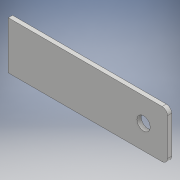
# Autodesk Inventor part: ramie3
Saved by Autodesk Inventor 2017.3 (Build 213256000, 256)
## iProperties
Created: 2019-03-17
Part Number: ramie3
Material: Ogólny
Document SubType Name: Modeling
Designer: legox
Density: 1 g/cm^3
Appearance: Domyślna
Author: legox
Autodesk Inventor part; units mm, degrees
ref_plane "YZ Plane" through (0, 0, 0) normal (1, 0, 0) x (0, 1, 0)
ref_plane "XZ Plane" through (0, 0, 0) normal (0, 1, 0) x (-1, 0, 0)
ref_plane "XY Plane" through (0, 0, 0) normal (0, 0, 1) x (1, 0, 0)
sketch "Szkic1" plane through (0, 0, 0) normal (0, 1, 0) x (-1, 0, 0)
  line L0 (2, 0) -> (60, 0)
  line L1 (60, 0) -> (60, -18)
  line L2 (60, -18) -> (2, -18)
  line L3 (0, -16) -> (0, -2)
  circle A0 centre (9, -9) radius 2.5
  arc A1 (0, -16) -> (2, -18) centre (2, -16) ccw
  arc A2 (2, 0) -> (0, -2) centre (2, -2) ccw
  point P0 (0, 0)
  point P1 (0, -18)
  dimension "d0" = 60
  dimension "d1" = 18
  dimension "d2" = 5
  dimension "d3" = 9
  dimension "d4" = 9
  dimension "d5" = 2
  constraints: 8 end point, 4 point on circle, 4 point on line, 4 tangent, 3 centre point, 2 parallel, 1 equal radius, 1 horizontal, 1 perpendicular
  measures "d0" distance of L1.end point (0, -18)
  measures "d1" distance of L0.end L1.end
  measures "d2" diameter of A0
  measures "d3" distance from line of L3 A0.centre
  measures "d4" distance from line of L0 A0.centre
  measures "d5" radius of A1
extrude "Wyciągnięcie proste1" add sketch "Szkic1" along normal blind 1.6
equation "\"d4\" = 0.5 * d1"
